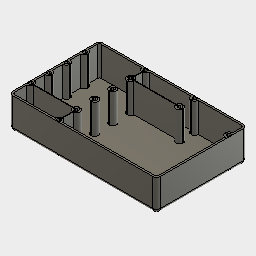
SIK_inserts v12 (Autodesk Fusion 360 design; units mm, degrees)
Autodesk Fusion 360 part; units mm, degrees
sketch "Sketch1" plane through (0, 0, 0) normal (0, 1, 0) x (1, 0, 0)
  line L0 (-107.65, -65.5) -> (133.65, -65.5)
  line L1 (140, -59.15) -> (140, 83.725)
  line L2 (133.65, 90.075) -> (-107.65, 90.075)
  line L3 (-114, 83.725) -> (-114, -59.15)
  arc A0 (-114, -59.15) -> (-107.65, -65.5) centre (-107.65, -59.15) ccw
  arc A1 (140, 83.725) -> (133.65, 90.075) centre (133.65, 83.725) ccw
  arc A2 (133.65, -65.5) -> (140, -59.15) centre (133.65, -59.15) ccw
  arc A3 (-107.65, 90.075) -> (-114, 83.725) centre (-107.65, 83.725) ccw
  point P0 (-114, -65.5)
  point P1 (140, -65.5)
  point P2 (-114, 90.075)
  dimension "d1" = 155.575
  dimension "d2" = 254
  dimension "d3" = 6.35
  dimension "d4" = 6.35
  dimension "d5" = 6.35
  dimension "d6" = 6.35
  measures "d1" distance of P0 P2
  measures "d2" distance of P0 P1
  measures "d3" radius of A0
  measures "d4" radius of A1
  measures "d5" radius of A2
  measures "d6" radius of A3
extrude "Extrude1" add sketch "Sketch1" along normal blind 3.175
sketch "Sketch2" plane through (0, 3.175, 0) normal (0, 1, 0) x (-1, 0, 0)
  arc A0 (107.65, -90.075) -> (114, -83.725) centre (107.65, -83.725) ccw
  line L0 (114, -83.725) -> (114, 59.15)
  arc A1 (114, 59.15) -> (107.65, 65.5) centre (107.65, 59.15) ccw
  line L1 (107.65, 65.5) -> (-133.65, 65.5)
  arc A2 (-133.65, 65.5) -> (-140, 59.15) centre (-133.65, 59.15) ccw
  line L2 (-140, 59.15) -> (-140, -83.725)
  arc A3 (-140, -83.725) -> (-133.65, -90.075) centre (-133.65, -83.725) ccw
  line L3 (-133.65, -90.075) -> (107.65, -90.075)
  line L4 (-136.825, 59.15) -> (-136.825, -83.725)
  arc A4 (-136.825, -83.725) -> (-133.65, -86.9) centre (-133.65, -83.725) ccw
  line L5 (-133.65, -86.9) -> (107.65, -86.9)
  arc A5 (107.65, -86.9) -> (110.825, -83.725) centre (107.65, -83.725) ccw
  line L6 (110.825, -83.725) -> (110.825, 59.15)
  arc A6 (110.825, 59.15) -> (107.65, 62.325) centre (107.65, 59.15) ccw
  line L7 (107.65, 62.325) -> (-133.65, 62.325)
  arc A7 (-133.65, 62.325) -> (-136.825, 59.15) centre (-133.65, 59.15) ccw
  circle A8 centre (31.45, 62.325) radius 3.175
  circle A9 centre (-136.825, -61.5) radius 3.175
  circle A10 centre (31.45, -61.5) radius 3.175
  circle A11 centre (31.45, -86.9) radius 3.175
  circle A12 centre (110.825, -61.5) radius 3.175
  circle A13 centre (31.45, 31.3688) radius 3.175
  circle A14 centre (31.45, 0.4125) radius 3.175
  circle A15 centre (31.45, -30.5437) radius 3.175
  circle A16 centre (-52.6875, -61.5) radius 3.175
  circle A17 centre (-52.6875, -86.9) radius 3.175
  circle A18 centre (110.825, -30.5437) radius 3.175
  circle A19 centre (110.825, 0.4125) radius 3.175
  circle A20 centre (110.825, 31.3688) radius 3.175
  circle A21 centre (31.45, 62.325) radius 6.35
  circle A22 centre (31.45, 31.3688) radius 6.35
  circle A23 centre (31.45, 0.4125) radius 6.35
  circle A24 centre (110.825, 31.3688) radius 6.35
  circle A25 centre (110.825, 0.4125) radius 6.35
  circle A26 centre (31.45, -30.5437) radius 6.35
  circle A27 centre (110.825, -30.5437) radius 6.35
  circle A28 centre (110.825, -61.5) radius 6.35
  circle A29 centre (31.45, -61.5) radius 6.35
  circle A30 centre (31.45, -86.9) radius 6.35
  circle A31 centre (-52.6875, -86.9) radius 6.35
  circle A32 centre (-52.6875, -61.5) radius 6.35
  circle A33 centre (-136.825, -61.5) radius 6.35
  line L8 (31.45, 31.3688) -> (110.825, 31.3688)
  line L9 (31.45, 0.4125) -> (110.825, 0.4125)
  line L10 (31.45, -30.5437) -> (110.825, -30.5437)
  line L11 (31.45, -61.5) -> (110.825, -61.5)
  line L12 (-52.6875, -61.5) -> (31.45, -61.5)
  line L13 (-136.825, -61.5) -> (-52.6875, -61.5)
  line L14 (-52.6875, -86.9) -> (-52.6875, -61.5)
  line L15 (31.45, -86.9) -> (31.45, -61.5)
  line L16 (31.45, -61.5) -> (31.45, -30.5437)
  line L17 (31.45, 0.4125) -> (31.45, -30.5437)
  line L18 (31.45, 31.3688) -> (31.45, 0.4125)
  line L19 (31.45, 62.325) -> (31.45, 31.3688)
  line L20 (31.45, 62.325) -> (31.45, 31.3688)
  line L21 (30.45, 62.325) -> (30.45, 31.3688)
  line L22 (31.45, 62.325) -> (31.45, 31.3688)
  line L23 (31.45, 62.325) -> (31.45, 31.3688)
  line L24 (32.45, 62.325) -> (32.45, 31.3688)
  line L25 (32.45, 31.3688) -> (32.45, 0.4125)
  line L26 (30.45, 31.3688) -> (30.45, 0.4125)
  line L27 (32.45, 0.4125) -> (32.45, -30.5437)
  line L28 (30.45, 0.4125) -> (30.45, -33.5572)
  line L29 (32.45, -30.5437) -> (32.45, -61.5)
  line L30 (30.45, -31.6976) -> (30.45, -61.5)
  line L31 (32.45, -61.5) -> (32.45, -86.9)
  line L32 (30.45, -61.5) -> (30.45, -86.9)
  line L33 (31.45, 30.3688) -> (110.825, 30.3688)
  line L34 (31.45, 31.3688) -> (110.825, 31.3688)
  line L35 (31.45, 32.3688) -> (110.825, 32.3688)
  line L36 (31.45, -0.5875) -> (110.825, -0.5875)
  line L37 (31.45, 0.4125) -> (110.825, 0.4125)
  line L38 (31.45, 1.4125) -> (110.825, 1.4125)
  line L39 (31.45, -31.5437) -> (110.825, -31.5437)
  line L40 (31.45, -30.5437) -> (110.825, -30.5437)
  line L41 (31.45, -29.5437) -> (110.825, -29.5437)
  line L42 (110.825, -61.5) -> (31.45, -61.5)
  line L43 (110.825, -60.5) -> (31.45, -60.5)
  line L44 (110.825, -62.5) -> (31.45, -62.5)
  line L45 (31.45, -62.5) -> (-136.825, -62.5)
  line L46 (31.45, -60.5) -> (-136.825, -60.5)
  line L47 (-52.6875, -61.5) -> (-52.6875, -86.9)
  line L48 (-51.6875, -86.9) -> (-51.6875, -61.5)
  line L49 (-53.6875, -86.9) -> (-53.6875, -61.5)
  line L50 (-133.65, -88.575) -> (107.65, -88.575)
  arc A34 (107.65, -88.575) -> (112.5, -83.725) centre (107.65, -83.725) ccw
  line L51 (112.5, -83.725) -> (112.5, 59.15)
  arc A35 (112.5, 59.15) -> (107.65, 64) centre (107.65, 59.15) ccw
  line L52 (107.65, 64) -> (-133.65, 64)
  arc A36 (-133.65, 64) -> (-138.5, 59.15) centre (-133.65, 59.15) ccw
  line L53 (-138.5, 59.15) -> (-138.5, -83.725)
  arc A37 (-138.5, -83.725) -> (-133.65, -88.575) centre (-133.65, -83.725) ccw
  line L54 (-136.825, -61.5) -> (-134.5799, -63.7451)
  line L55 (-136.825, -61.5) -> (-133.65, -61.5) construction
  line L56 (-136.825, -61.5) -> (-139.0701, -59.2549)
  line L57 (-136.825, -61.5) -> (-133.65, -61.5) construction
  line L58 (-136.825, -61.5) -> (-139.0701, -63.7451)
  line L59 (-136.825, -61.5) -> (-134.5799, -59.2549)
  line L60 (-136.4714, -61.8536) -> (-134.2264, -59.6085)
  line L61 (-136.4714, -61.8536) -> (-138.7165, -64.0986)
  line L62 (-139.0701, -63.7451) -> (-134.5799, -59.2549)
  line L63 (-139.4236, -63.3915) -> (-134.9335, -58.9014)
  line L64 (-136.4714, -61.1464) -> (-134.2264, -63.3915)
  line L65 (-136.4714, -61.1464) -> (-138.7165, -58.9014)
  line L66 (-134.5799, -63.7451) -> (-139.0701, -59.2549)
  line L67 (-134.9335, -64.0986) -> (-139.4236, -59.6085)
  line L68 (-136.4714, -61.8536) -> (-138.7165, -64.0986)
  line L69 (-139.4236, -63.3915) -> (-134.9335, -58.9014)
  line L70 (-136.4714, -61.1464) -> (-138.7165, -58.9014)
  line L71 (-136.4714, -61.8536) -> (-134.2264, -59.6085)
  line L72 (-136.4714, -61.1464) -> (-134.2264, -63.3915)
  circle A38 centre (-136.825, -61.5) radius 3.175
  line L73 (-50.796, -64.0986) -> (-55.2861, -59.6085)
  line L74 (-52.3339, -61.1464) -> (-54.579, -58.9014)
  line L75 (-52.3339, -61.1464) -> (-50.0889, -63.3915)
  line L76 (-52.3339, -61.8536) -> (-54.579, -64.0986)
  line L77 (-55.2861, -63.3915) -> (-50.796, -58.9014)
  line L78 (-52.3339, -61.8536) -> (-50.0889, -59.6085)
  circle A39 centre (-52.6875, -61.5) radius 3.175
  line L79 (-55.2861, -88.7915) -> (-50.796, -84.3014)
  line L80 (-52.3339, -87.2536) -> (-54.579, -89.4986)
  circle A40 centre (-52.6875, -86.9) radius 3.175
  line L81 (-50.796, -89.4986) -> (-55.2861, -85.0085)
  line L82 (-52.3339, -86.5464) -> (-50.0889, -88.7915)
  line L83 (-52.3339, -87.2536) -> (-50.0889, -85.0085)
  line L84 (-52.3339, -86.5464) -> (-54.579, -84.3014)
  line L85 (28.8514, -63.3915) -> (33.3415, -58.9014)
  line L86 (31.8036, -61.8536) -> (29.5585, -64.0986)
  circle A41 centre (31.45, -61.5) radius 3.175
  line L87 (33.3415, -64.0986) -> (28.8514, -59.6085)
  line L88 (31.8036, -61.1464) -> (34.0486, -63.3915)
  line L89 (31.8036, -61.8536) -> (34.0486, -59.6085)
  line L90 (31.8036, -61.1464) -> (29.5585, -58.9014)
  line L91 (28.8514, -88.7915) -> (33.3415, -84.3014)
  line L92 (31.8036, -87.2536) -> (29.5585, -89.4986)
  circle A42 centre (31.45, -86.9) radius 3.175
  line L93 (33.3415, -89.4986) -> (28.8514, -85.0085)
  line L94 (31.8036, -86.5464) -> (34.0486, -88.7915)
  line L95 (31.8036, -87.2536) -> (34.0486, -85.0085)
  line L96 (31.8036, -86.5464) -> (29.5585, -84.3014)
  line L97 (108.2264, -63.3915) -> (112.7165, -58.9014)
  line L98 (111.1786, -61.8536) -> (108.9335, -64.0986)
  circle A43 centre (110.825, -61.5) radius 3.175
  line L99 (112.7165, -64.0986) -> (108.2264, -59.6085)
  line L100 (111.1786, -61.1464) -> (113.4236, -63.3915)
  line L101 (111.1786, -61.8536) -> (113.4236, -59.6085)
  line L102 (111.1786, -61.1464) -> (108.9335, -58.9014)
  line L103 (28.8514, -32.4353) -> (33.3415, -27.9451)
  line L104 (31.8036, -30.8973) -> (29.5585, -33.1424)
  circle A44 centre (31.45, -30.5437) radius 3.175
  line L105 (33.3415, -33.1424) -> (28.8514, -28.6522)
  line L106 (31.8036, -30.1902) -> (34.0486, -32.4353)
  line L107 (31.8036, -30.8973) -> (34.0486, -28.6522)
  line L108 (31.8036, -30.1902) -> (29.5585, -27.9451)
  line L109 (28.8514, -1.479) -> (33.3415, 3.0111)
  line L110 (31.8036, 0.0589) -> (29.5585, -2.1861)
  circle A45 centre (31.45, 0.4125) radius 3.175
  line L111 (33.3415, -2.1861) -> (28.8514, 2.304)
  line L112 (31.8036, 0.7661) -> (34.0486, -1.479)
  line L113 (31.8036, 0.0589) -> (34.0486, 2.304)
  line L114 (31.8036, 0.7661) -> (29.5585, 3.0111)
  line L115 (108.2264, -32.4353) -> (112.7165, -27.9451)
  line L116 (111.1786, -30.8973) -> (108.9335, -33.1424)
  circle A46 centre (110.825, -30.5437) radius 3.175
  line L117 (112.7165, -33.1424) -> (108.2264, -28.6522)
  line L118 (111.1786, -30.1902) -> (113.4236, -32.4353)
  line L119 (111.1786, -30.8973) -> (113.4236, -28.6522)
  line L120 (111.1786, -30.1902) -> (108.9335, -27.9451)
  line L121 (108.2264, -1.479) -> (112.7165, 3.0111)
  line L122 (111.1786, 0.0589) -> (108.9335, -2.1861)
  circle A47 centre (110.825, 0.4125) radius 3.175
  line L123 (112.7165, -2.1861) -> (108.2264, 2.304)
  line L124 (111.1786, 0.7661) -> (113.4236, -1.479)
  line L125 (111.1786, 0.0589) -> (113.4236, 2.304)
  line L126 (111.1786, 0.7661) -> (108.9335, 3.0111)
  line L127 (28.8514, 29.4772) -> (33.3415, 33.9674)
  line L128 (31.8036, 31.0152) -> (29.5585, 28.7701)
  circle A48 centre (31.45, 31.3688) radius 3.175
  line L129 (33.3415, 28.7701) -> (28.8514, 33.2603)
  line L130 (31.8036, 31.7223) -> (34.0486, 29.4772)
  line L131 (31.8036, 31.0152) -> (34.0486, 33.2603)
  line L132 (31.8036, 31.7223) -> (29.5585, 33.9674)
  line L133 (108.2264, 29.4772) -> (112.7165, 33.9674)
  line L134 (111.1786, 31.0152) -> (108.9335, 28.7701)
  circle A49 centre (110.825, 31.3688) radius 3.175
  line L135 (112.7165, 28.7701) -> (108.2264, 33.2603)
  line L136 (111.1786, 31.7223) -> (113.4236, 29.4772)
  line L137 (111.1786, 31.0152) -> (113.4236, 33.2603)
  line L138 (111.1786, 31.7223) -> (108.9335, 33.9674)
  line L139 (28.8514, 60.4335) -> (33.3415, 64.9236)
  line L140 (31.8036, 61.9714) -> (29.5585, 59.7264)
  circle A50 centre (31.45, 62.325) radius 3.175
  line L141 (33.3415, 59.7264) -> (28.8514, 64.2165)
  line L142 (31.8036, 62.6786) -> (34.0486, 60.4335)
  line L143 (31.8036, 61.9714) -> (34.0486, 64.2165)
  line L144 (31.8036, 62.6786) -> (29.5585, 64.9236)
  point P0 (31.45, -61.5)
  dimension "d9" = 3.175
  dimension "d12" = 165.1
  dimension "d13" = 120.65
  dimension "d14" = 6.35
  dimension "d15" = 6.35
  dimension "d18" = 6.35
  dimension "d19" = 6.35
  dimension "d20" = 6.35
  dimension "d21" = 6.35
  dimension "d22" = 6.35
  dimension "d23" = 6.35
  dimension "d24" = 6.35
  dimension "d25" = 6.35
  dimension "d26" = 6.35
  dimension "d27" = 6.35
  dimension "d28" = 6.35
  dimension "d29" = 3.175
  dimension "d30" = 3.175
  dimension "d31" = 3.175
  dimension "d32" = 3.175
  dimension "d33" = 3.175
  dimension "d34" = 3.175
  dimension "d35" = 3.175
  dimension "d36" = 3.175
  dimension "d37" = 3.175
  dimension "d38" = 3.175
  dimension "d39" = 3.175
  dimension "d40" = 3.175
  dimension "d41" = 3.175
  dimension "d42" = 1
  dimension "d43" = 1
  dimension "d44" = 1
  dimension "d45" = 1
  dimension "d46" = 1
  dimension "d47" = 1
  dimension "d48" = 1
  dimension "d49" = 1
  dimension "d50" = 1
  dimension "d51" = 1
  dimension "d52" = 1
  dimension "d53" = 1
  dimension "d54" = 1.5
  dimension "d58" = 45
  dimension "d59" = 135
  dimension "d60" = 0.5
  dimension "d61" = 0.5
  dimension "d62" = 0.5
  dimension "d63" = 0.5
  dimension "d64" = 6.35
  dimension "d65" = 6.35
  dimension "d66" = 6.35
  dimension "d67" = 6.35
  dimension "d68" = 6.35
  dimension "d69" = 6.35
  dimension "d70" = 6.35
  dimension "d71" = 6.35
  dimension "d72" = 6.35
  dimension "d73" = 6.35
  dimension "d74" = 6.35
  dimension "d75" = 6.35
  dimension "d76" = 6.35
  measures "d12" distance of L7.end A8.centre
  measures "d13" distance of L4.start A9.centre
  measures "d14" diameter of A8
  measures "d15" diameter of A9
  measures "d18" diameter of A10
  measures "d19" diameter of A11
  measures "d20" diameter of A12
  measures "d21" diameter of A13
  measures "d22" diameter of A14
  measures "d23" diameter of A15
  measures "d24" diameter of A16
  measures "d25" diameter of A17
  measures "d26" diameter of A18
  measures "d27" diameter of A19
  measures "d28" diameter of A20
  measures "d29" distance of A8
  measures "d30" distance of A13
  measures "d31" distance of A14
  measures "d32" distance of A20
  measures "d33" distance of A19
  measures "d34" distance of A15
  measures "d35" distance of A18
  measures "d36" distance of A12
  measures "d37" distance of A10
  measures "d38" distance of A11
  measures "d39" distance of A17
  measures "d40" distance of A16
  measures "d41" distance of A9
  measures "d58" angle of L54 L55
  measures "d59" angle of L56 L57
  measures "d64" diameter of A38
  measures "d65" diameter of A39
  measures "d66" diameter of A40
  measures "d67" diameter of A41
  measures "d68" diameter of A42
  measures "d69" diameter of A43
  measures "d70" diameter of A44
  measures "d71" diameter of A45
  measures "d72" diameter of A46
  measures "d73" diameter of A47
  measures "d74" diameter of A48
  measures "d75" diameter of A49
  measures "d76" diameter of A50
extrude "Extrude2" add sketch "Sketch2" along normal blind 50.8 contours A0 L0 L3 A28 A30 L50 A34 L51 | L3 A11 A30 L50 A42 | L0 A12 A28 L51 A43 | L3 A11 A30 L50 A42 | A11 L50 L92 A42 L93 | L3 A30 A31 L50 | L5 A11 A30 L50 A42 | L5 A5 L6 A28 A30 L50 A34 L51 | L0 A12 A28 L51 A43 | A12 L51 A43 L100 L101 | L6 A12 A28 L51 A43 | A11 L50 L91 L92 A42 | A11 L50 A42 L93 L94 | L3 A17 A31 L50 A40 | L5 A30 A31 L50 | L5 A11 A30 L50 A42 | L5 A11 A30 L31 A42 | A11 L50 A42 L94 | L0 A27 A28 L51 | A12 L51 L97 A43 L101 | A12 L51 A43 L99 L100 | L6 A12 A28 L44 A43 | A12 L51 A43 L99 | A11 L50 L91 A42 | L3 A17 A31 L50 A40 | A17 L50 L80 A40 L81 | L2 A3 L3 A31 A33 L50 L53 A37 | L5 A17 A31 L50 A40 | L5 A11 A30 L32 A42 | L0 A18 A27 L51 A46 | L6 A12 A28 L51 A43 | L6 A27 A28 L51 | A12 L51 L97 A43 | A17 L50 L79 L80 A40 | A17 L50 A40 L81 L82 | L4 A4 L5 A31 A33 L50 L53 A37 | L5 A17 A31 L50 A40 | L5 A17 A31 L48 A40 | A17 L50 A40 L82 | A10 A29 L31 L44 A41 | L0 A18 A27 L51 A46 | A18 L51 A46 L118 L119 | L6 A18 A27 L51 A46 | L6 A12 A28 L43 A43 | A17 L50 L79 A40 | L5 A17 A31 L49 A40 | A10 A29 L32 L45 A41 | L0 A25 A27 L51 | A18 L51 L115 A46 L119 | A18 L51 A46 L117 L118 | L6 A18 A27 L39 A46 | A18 L51 A46 L117 | L2 A9 A33 L53 A38 | A16 A32 L45 L48 A39 | L0 A19 A25 L51 A47 | L6 A18 A27 L51 A46 | L6 A25 A27 L51 | A18 L51 L115 A46 | A10 A29 L29 L43 A41 | L2 A9 A33 L53 A38 | A9 L53 L63 L67 L69 A38 | L1 A2 L2 A21 A33 L52 A36 L53 | L4 A9 A33 L53 A38 | A16 A32 L45 L49 A39 | L0 A19 A25 L51 A47 | A19 L51 A47 L124 L125 | L6 A19 A25 L51 A47 | L6 A18 A27 L41 A46 | A15 A26 L29 L39 A44 | A9 L53 L56 L66 L67 A38 | A9 L53 L58 L62 L63 L69 A38 | L4 L7 A7 A21 A33 L52 A36 L53 | L4 A9 A33 L53 A38 | L4 A9 A33 L45 A38 | A9 L53 L61 L68 A38 | A10 A29 L30 L46 A41 | L0 A24 A25 L51 | A19 L51 L121 A47 L125 | A19 L51 A47 L123 L124 | L6 A19 A25 L36 A47 | A19 L51 A47 L123 | A9 L53 L56 L65 L66 L70 A38 | A9 L53 L58 L61 L62 L68 A38 | L4 A9 A33 L46 A38 | A9 L53 L65 L70 A38 | A16 A32 L46 A39 | L0 A20 A24 L51 A49 | L6 A19 A25 L51 A47 | L6 A24 A25 L51 | A19 L51 L121 A47 | A15 A26 L27 L41 A44 | L1 A8 A21 L52 A50 | A15 A26 L28 L30 A44 | L0 A20 A24 L51 A49 | A20 L51 A49 L136 L137 | L6 A20 A24 L51 A49 | L6 A19 A25 L38 A47 | A14 A23 L27 L36 A45 | L1 A8 A21 L52 A50 | A8 L52 L139 A50 L144 | L0 A1 L1 A21 A24 L51 A35 L52 | L7 A8 A21 L52 A50 | A20 L51 L133 A49 L137 | A20 L51 A49 L135 L136 | L6 A20 A24 L33 A49 | A20 L51 A49 L135 | A8 L52 L139 A50 L143 | A8 L52 A50 L141 L144 | L6 A6 L7 A21 A24 L51 A35 L52 | L7 A8 A21 L52 A50 | L7 A8 A21 L21 A50 | A8 L52 A50 L141 | A14 A23 L26 L28 A45 | L6 A20 A24 L51 A49 | A20 L51 L133 A49 | A14 A23 L25 L38 A45 | A8 L52 A50 L143 | L7 A8 A21 L24 A50 | L6 A20 A24 L35 A49 | A13 A22 L25 L33 A48 | A13 A22 L21 L26 A48 | A13 A22 L24 L35 A48
fillet "Fillet1" radius 6.35 8 edges at (140, 0, -12.2875) (138.1401, 0, -88.2151) (13, 0, -90.075) (-112.1401, 0, -88.2151) (-114, 0, -12.2875) (-112.1401, 0, 63.6401) (13, 0, 65.5) (138.1401, 0, 63.6401)
sketch "split_break_dividers" plane through (0, 3.175, -3.175) normal (0, 1, 0) x (1, 0, 0)
  arc A0 (-32.45, -28.273) -> (-37.7208, -33.5438) centre (-31.45, -34.5438) ccw
  line L0 (50.6268, 57.6786) -> (50.226, 57.2777)
  arc A1 (50.226, 57.2777) -> (50.0596, 57.825) centre (52.6875, 58.325) cw
  line L1 (-107.65, 83.725) -> (133.65, 83.725)
  line L2 (134.5799, 60.5701) -> (139.0701, 56.0799)
  line L3 (-111.1786, 27.0152) -> (-108.9335, 24.7701)
  line L4 (136.4714, 58.6786) -> (134.2264, 56.4335)
  line L5 (-31.8036, 58.6786) -> (-34.0486, 56.4335)
  line L6 (-31.8036, 57.9714) -> (-34.0486, 60.2165)
  line L7 (52.3339, 83.3714) -> (54.579, 81.1264)
  line L8 (136.4714, 58.6786) -> (134.2264, 56.4335)
  line L9 (133.65, -67.175) -> (-107.65, -67.175)
  line L10 (-31.8036, -3.9411) -> (-29.5585, -6.1861)
  line L11 (51.2733, 58.325) -> (50.6268, 57.6786)
  line L12 (-28.8514, -1.696) -> (-33.3415, -6.1861)
  line L13 (-31.8036, 27.0152) -> (-34.0486, 29.2603)
  line L14 (-112.5, -62.325) -> (-112.5, 80.55)
  line L15 (-107.65, 86.9) -> (133.65, 86.9)
  arc A2 (136.825, -62.325) -> (133.65, -65.5) centre (133.65, -62.325) cw
  arc A3 (-28.8221, 57.825) -> (-28.9885, 57.2777) centre (-31.45, 58.325) cw
  line L16 (55.2861, 60.2165) -> (50.796, 55.7264)
  line L17 (-31.8036, 27.0152) -> (-29.5585, 24.7701)
  line L18 (-31.8036, -3.2339) -> (-29.5585, -0.9889)
  line L19 (140, 80.55) -> (140, -62.325)
  line L20 (-114, -62.325) -> (-114, 80.55)
  arc A4 (-107.65, -65.5) -> (-110.825, -62.325) centre (-107.65, -62.325) cw
  line L21 (-108.2264, 29.2603) -> (-112.7165, 24.7701)
  line L22 (50.796, 60.9236) -> (55.2861, 56.4335)
  line L23 (52.3339, 83.3714) -> (50.0889, 85.6165)
  line L24 (-31.8036, -3.2339) -> (-34.0486, -5.479)
  line L25 (133.65, -65.5) -> (-107.65, -65.5)
  line L26 (-33.3415, 29.9674) -> (-28.8514, 25.4772)
  line L27 (133.65, -68.675) -> (-107.65, -68.675)
  line L28 (-31.8036, 27.7223) -> (-34.0486, 25.4772)
  line L29 (-31.8036, -3.9411) -> (-34.0486, -1.696)
  line L30 (-33.3415, -0.9889) -> (-28.8514, -5.479)
  line L31 (55.2861, 85.6165) -> (50.796, 81.1264)
  line L32 (136.4714, 57.9714) -> (134.2264, 60.2165)
  line L33 (-107.65, 85.4) -> (133.65, 85.4)
  arc A5 (-107.65, -67.175) -> (-112.5, -62.325) centre (-107.65, -62.325) cw
  arc A6 (133.65, 83.725) -> (136.825, 80.55) centre (133.65, 80.55) cw
  arc A7 (-110.825, 80.55) -> (-107.65, 83.725) centre (-107.65, 80.55) cw
  line L34 (136.825, 80.55) -> (136.825, -62.325)
  arc A8 (140, -62.325) -> (133.65, -68.675) centre (133.65, -62.325) cw
  line L35 (52.3339, 58.6786) -> (54.579, 60.9236)
  line L36 (-111.1786, 27.7223) -> (-113.4236, 25.4772)
  line L37 (-111.1786, 58.6786) -> (-113.4236, 56.4335)
  line L38 (136.825, 58.325) -> (134.5799, 60.5701)
  line L39 (-110.825, -62.325) -> (-110.825, 80.55)
  arc A9 (-114, 80.55) -> (-107.65, 86.9) centre (-107.65, 80.55) cw
  line L40 (136.825, 58.325) -> (136.1179, 58.325)
  arc A10 (-107.65, -68.675) -> (-114, -62.325) centre (-107.65, -62.325) cw
  line L41 (136.4714, 57.9714) -> (134.2264, 60.2165)
  arc A11 (-112.5, 80.55) -> (-107.65, 85.4) centre (-107.65, 80.55) cw
  line L42 (50.6268, 58.9714) -> (51.2733, 58.325)
  line L43 (52.3339, 57.9714) -> (54.579, 55.7264)
  line L44 (-112.7165, 60.9236) -> (-108.2264, 56.4335)
  arc A12 (138.5, -62.325) -> (133.65, -67.175) centre (133.65, -62.325) cw
  line L45 (138.5, 80.55) -> (138.5, -62.325)
  line L46 (50.0596, 57.825) -> (-28.8221, 57.825)
  line L47 (136.4714, 57.9714) -> (138.7165, 55.7264)
  arc A13 (133.65, 85.4) -> (138.5, 80.55) centre (133.65, 80.55) cw
  arc A14 (133.65, 86.9) -> (140, 80.55) centre (133.65, 80.55) cw
  line L48 (-111.1786, 27.7223) -> (-108.9335, 29.9674)
  line L49 (139.0701, 60.5701) -> (134.5799, 56.0799)
  line L50 (-111.1786, 27.0152) -> (-113.4236, 29.2603)
  arc A15 (-34.0779, -35.0438) -> (-33.9115, -35.591) centre (-31.45, -34.5438) ccw
  line L51 (-109.1179, -33.5438) -> (-110.1179, -34.5438)
  line L52 (-29.5865, 60.8956) -> (-29.5585, 60.9236)
  line L53 (-34.0206, -36.4072) -> (-34.0486, -36.4353)
  line L54 (-108.1971, -35.0438) -> (-34.0779, -35.0438)
  line L55 (-30.45, 60.0321) -> (-29.5865, 60.8956)
  line L56 (-33.3415, 60.9236) -> (-33.3135, 60.8956)
  line L57 (-33.5107, -33.8973) -> (-33.9115, -33.4965)
  line L58 (-33.3135, -31.9731) -> (-31.45, -33.8366)
  line L59 (-31.45, -33.8366) -> (-28.8514, -36.4353)
  line L60 (-33.1571, -33.5438) -> (-34.0206, -32.6803)
  line L61 (-32.8642, -34.5438) -> (-33.5107, -33.8973)
  line L62 (-33.1571, -35.5438) -> (-34.0206, -36.4072)
  line L63 (-33.5107, -35.1902) -> (-32.8642, -34.5438)
  line L64 (-31.1571, 59.325) -> (-30.45, 60.0321)
  line L65 (50.1169, 60.1885) -> (50.0889, 60.2165)
  line L66 (50.9804, 59.325) -> (50.1169, 60.1885)
  line L67 (51.6875, 58.6179) -> (50.9804, 59.325)
  arc A16 (49.6741, 57.325) -> (50.1169, 56.4615) centre (52.6875, 58.325) ccw
  line L68 (-32.45, 82.0179) -> (-33.3135, 81.1544)
  arc A17 (50.1169, 60.1885) -> (49.6741, 59.325) centre (52.6875, 58.325) ccw
  line L69 (-28.9885, 57.2777) -> (-29.3893, 57.6786)
  line L70 (-28.8794, 56.4615) -> (-28.8514, 56.4335)
  line L71 (-110.1179, -34.5438) -> (-112.7165, -37.1424)
  line L72 (-108.2544, -36.4072) -> (-108.2264, -36.4353)
  line L73 (-108.2264, -32.6522) -> (-108.2544, -32.6803)
  line L74 (-112.7165, -31.9451) -> (-110.1179, -34.5438)
  arc A18 (-107.8116, -33.5438) -> (-108.2544, -32.6803) centre (-110.825, -34.5438) ccw
  arc A19 (-34.4634, -35.5438) -> (-34.0206, -36.4072) centre (-31.45, -34.5438) ccw
  arc A20 (-108.3635, -35.591) -> (-108.1971, -35.0438) centre (-110.825, -34.5438) ccw
  line L75 (-34.0206, -32.6803) -> (-34.0486, -32.6522)
  line L76 (-33.9115, -35.591) -> (-33.5107, -35.1902)
  arc A21 (-33.9115, -33.4965) -> (-34.0779, -34.0438) centre (-31.45, -34.5438) ccw
  arc A22 (-32.45, -31.5303) -> (-33.3135, -31.9731) centre (-31.45, -34.5438) ccw
  line L77 (-108.2544, -32.6803) -> (-109.1179, -33.5438)
  line L78 (-108.7643, -35.1902) -> (-108.3635, -35.591)
  line L79 (-30.7429, 58.325) -> (-30.45, 58.0321)
  arc A23 (-32.4973, 60.7865) -> (-31.95, 60.9529) centre (-31.45, 58.325) cw
  arc A24 (-108.1971, -34.0438) -> (-108.3635, -33.4965) centre (-110.825, -34.5438) ccw
  line L80 (-110.1179, -34.5438) -> (-109.1179, -35.5438)
  line L81 (-109.1179, -35.5438) -> (-108.2544, -36.4072)
  line L82 (-34.0779, -34.0438) -> (-108.1971, -34.0438)
  line L83 (-32.45, -34.2509) -> (-33.1571, -33.5438)
  line L84 (-108.3635, -33.4965) -> (-108.7643, -33.8973)
  line L85 (-109.4108, -34.5438) -> (-108.7643, -35.1902)
  arc A25 (-108.2544, -36.4072) -> (-107.8116, -35.5438) centre (-110.825, -34.5438) ccw
  line L86 (-33.3415, -31.9451) -> (-33.3135, -31.9731)
  line L87 (-32.45, -34.8366) -> (-33.1571, -35.5438)
  line L88 (-108.7643, -33.8973) -> (-109.4108, -34.5438)
  line L89 (51.9804, 58.325) -> (50.9804, 57.325)
  line L90 (-33.3135, 81.1544) -> (-33.3415, 81.1264)
  line L91 (-31.45, 83.0179) -> (-32.45, 82.0179)
  arc A26 (-33.3135, 81.1544) -> (-32.45, 80.7116) centre (-31.45, 83.725) ccw
  line L92 (-30.0358, 58.325) -> (-29.3893, 58.9714)
  arc A27 (50.0596, 58.825) -> (50.226, 59.3723) centre (52.6875, 58.325) cw
  line L93 (-30.4027, 60.7865) -> (-30.8036, 60.3857)
  line L94 (50.9804, 57.325) -> (50.1169, 56.4615)
  line L95 (-31.8036, 83.3714) -> (-31.45, 83.0179)
  line L96 (52.3339, 57.9714) -> (51.9804, 58.325)
  line L97 (-30.45, 82.0179) -> (-29.5865, 81.1544)
  line L98 (50.226, 59.3723) -> (50.6268, 58.9714)
  line L99 (-28.8794, 60.1885) -> (-29.7429, 59.325)
  line L100 (-30.8036, 60.3857) -> (-31.45, 59.7392)
  line L101 (-31.95, 60.9529) -> (-31.95, 81.0971)
  arc A28 (-28.4366, 59.325) -> (-28.8794, 60.1885) centre (-31.45, 58.325) ccw
  line L102 (-31.45, 82.3108) -> (-30.8036, 81.6643)
  line L103 (-29.7429, 59.325) -> (-30.45, 58.6179)
  line L104 (-32.4973, 81.2635) -> (-32.0964, 81.6643)
  arc A29 (-30.4027, 81.2635) -> (-30.95, 81.0971) centre (-31.45, 83.725) cw
  line L105 (-29.5865, 81.1544) -> (-29.5585, 81.1264)
  line L106 (-33.3135, 60.8956) -> (-32.45, 60.0321)
  line L107 (-31.7429, 59.325) -> (-31.45, 59.0321)
  line L108 (-31.45, 59.0321) -> (-30.7429, 58.325)
  arc A30 (-29.5865, 60.8956) -> (-30.45, 61.3384) centre (-31.45, 58.325) ccw
  line L109 (-28.8514, 60.2165) -> (-28.8794, 60.1885)
  line L110 (-28.8514, 85.6165) -> (-31.45, 83.0179)
  arc A31 (-32.45, 61.3384) -> (-33.3135, 60.8956) centre (-31.45, 58.325) ccw
  arc A32 (-31.95, 81.0971) -> (-32.4973, 81.2635) centre (-31.45, 83.725) cw
  line L111 (-30.8036, 81.6643) -> (-30.4027, 81.2635)
  line L112 (51.9804, 58.325) -> (51.6875, 58.6179)
  line L113 (-29.3893, 57.6786) -> (-30.0358, 58.325)
  line L114 (-31.45, 59.7392) -> (-32.0964, 60.3857)
  line L115 (-29.7429, 57.325) -> (-28.8794, 56.4615)
  arc A33 (-28.8794, 56.4615) -> (-28.4366, 57.325) centre (-31.45, 58.325) ccw
  line L116 (-30.45, 58.0321) -> (-29.7429, 57.325)
  line L117 (-32.45, 60.0321) -> (-31.7429, 59.325)
  arc A34 (-30.95, 60.9529) -> (-30.4027, 60.7865) centre (-31.45, 58.325) cw
  line L118 (-31.45, 83.0179) -> (-30.45, 82.0179)
  line L119 (-31.45, 59.0321) -> (-31.1571, 59.325)
  line L120 (-32.0964, 81.6643) -> (-31.45, 82.3108)
  line L121 (-32.0964, 60.3857) -> (-32.4973, 60.7865)
  line L122 (52.3339, 58.6786) -> (51.9804, 58.325)
  arc A35 (-28.9885, 59.3723) -> (-28.8221, 58.825) centre (-31.45, 58.325) cw
  line L123 (-28.8221, 58.825) -> (50.0596, 58.825)
  line L124 (-29.3893, 58.9714) -> (-28.9885, 59.3723)
  line L125 (-31.8036, 58.6786) -> (-31.45, 59.0321)
  line L126 (-30.7429, 58.325) -> (-33.3415, 55.7264)
  arc A36 (-30.45, 80.7116) -> (-29.5865, 81.1544) centre (-31.45, 83.725) ccw
  line L127 (50.1169, 56.4615) -> (50.0889, 56.4335)
  line L128 (-30.45, 58.6179) -> (-30.7429, 58.325)
  line L129 (-30.95, 81.0971) -> (-30.95, 60.9529)
  line L130 (-31.45, -34.5438) -> (-32.1571, -34.5438)
  line L131 (-34.4634, -2.5875) -> (-107.8116, -2.5875)
  line L132 (-110.825, 58.325) -> (-110.1179, 58.325)
  line L133 (-34.4634, -35.5438) -> (-107.8116, -35.5438)
  arc A37 (-32.45, 33.6395) -> (-37.7208, 28.3687) centre (-31.45, 27.3687) ccw
  line L134 (-31.7429, -2.5875) -> (-33.1571, -2.5875)
  line L135 (-34.4634, 26.3687) -> (-107.8116, 26.3687)
  arc A38 (-37.7208, 26.3687) -> (-30.45, 33.6395) centre (-31.45, 27.3687) ccw
  line L136 (-32.45, -35.5438) -> (-33.1571, -35.5438)
  line L137 (-110.825, 59.325) -> (-109.1179, 59.325)
  arc A39 (-34.4634, -4.5875) -> (-32.45, -6.6009) centre (-31.45, -3.5875) ccw
  line L138 (-31.45, -3.5875) -> (-32.1571, -3.5875)
  arc A40 (-37.7208, -35.5438) -> (-32.45, -40.8145) centre (-31.45, -34.5438) ccw
  arc A41 (-107.8116, -2.5875) -> (-107.8116, -4.5875) centre (-110.825, -3.5875) ccw
  line L139 (-109.1179, -4.5875) -> (-110.825, -4.5875)
  arc A42 (-30.45, 80.7116) -> (-33.3135, 81.1544) centre (-31.45, 83.725) ccw
  arc A43 (-33.3135, -31.9731) -> (-34.0206, -32.6803) centre (-31.45, -34.5438) ccw
  line L140 (-32.45, -33.5438) -> (-33.1571, -33.5438)
  line L141 (-31.7429, 28.3687) -> (-33.1571, 28.3687)
  arc A44 (-34.4634, 26.3687) -> (-32.45, 24.3553) centre (-31.45, 27.3687) ccw
  arc A45 (-104.5542, 28.3687) -> (-104.5542, 26.3687) centre (-110.825, 27.3687) ccw
  line L142 (-34.4634, -33.5438) -> (-107.8116, -33.5438)
  arc A46 (-34.0206, -36.4072) -> (-33.3135, -37.1144) centre (-31.45, -34.5438) ccw
  arc A47 (-32.45, 2.6833) -> (-37.7208, -2.5875) centre (-31.45, -3.5875) ccw
  line L143 (-31.45, 27.3687) -> (-32.1571, 27.3687)
  arc A48 (-34.4634, 26.3687) -> (-32.45, 24.3553) centre (-31.45, 27.3687) ccw
  line L144 (-110.1179, 58.325) -> (-110.825, 58.325)
  line L145 (-31.45, -3.5875) -> (-32.1571, -3.5875)
  arc A49 (-29.5865, 81.1544) -> (-32.45, 80.7116) centre (-31.45, 83.725) ccw
  line L146 (-32.45, 82.0179) -> (-32.45, 83.725)
  line L147 (-109.1179, -33.5438) -> (-110.825, -33.5438)
  line L148 (-34.4634, -4.5875) -> (-107.8116, -4.5875)
  line L149 (-30.45, -62.4866) -> (-30.45, -37.5572)
  line L150 (-30.45, 56.6179) -> (-30.45, 58.0321)
  line L151 (-32.45, 30.3822) -> (-32.45, 55.3116)
  arc A50 (-30.45, -6.6009) -> (-30.45, -0.5741) centre (-31.45, -3.5875) ccw
  arc A51 (-30.45, -9.8583) -> (-30.45, 2.6833) centre (-31.45, -3.5875) ccw
  line L152 (-32.45, -62.4866) -> (-32.45, -37.5572)
  arc A52 (-30.45, -37.5572) -> (-30.45, -31.5303) centre (-31.45, -34.5438) ccw
  line L153 (-31.45, -3.5875) -> (-31.45, -2.8804)
  line L154 (-32.45, 27.6616) -> (-32.45, 29.0759)
  line L155 (-112.7165, -0.9889) -> (-108.2264, -5.479)
  arc A53 (-30.45, 24.3553) -> (-30.45, 30.3822) centre (-31.45, 27.3687) ccw
  line L156 (-111.1786, -34.8973) -> (-113.4236, -32.6522)
  line L157 (-111.1786, -3.9411) -> (-113.4236, -1.696)
  line L158 (-30.45, 28.5226) -> (-30.45, 29.0759)
  arc A54 (-33.3135, -62.9294) -> (-29.5865, -62.9294) centre (-31.45, -65.5) ccw
  line L159 (-31.8036, -65.8536) -> (-34.0486, -63.6085)
  line L160 (-32.45, 25.6616) -> (-32.45, 27.0759)
  arc A55 (-29.5865, -37.1144) -> (-29.5865, -31.9731) centre (-31.45, -34.5438) ccw
  line L161 (-32.45, 56.6179) -> (-32.45, 58.0321)
  arc A56 (-32.45, 30.3822) -> (-34.4634, 28.3687) centre (-31.45, 27.3687) ccw
  line L162 (-31.45, 59.0321) -> (-31.45, 58.325)
  line L163 (-112.7165, 29.9674) -> (-108.2264, 25.4772)
  line L164 (-111.1786, 57.9714) -> (-113.4236, 60.2165)
  line L165 (-33.3415, 86.3236) -> (-28.8514, 81.8335)
  line L166 (52.3339, 84.0786) -> (50.0889, 81.8335)
  line L167 (-31.8036, 57.9714) -> (-29.5585, 55.7264)
  line L168 (52.3339, 84.0786) -> (54.579, 86.3236)
  line L169 (-31.8036, 84.0786) -> (-34.0486, 81.8335)
  line L170 (134.9335, 60.9236) -> (139.4236, 56.4335)
  line L171 (136.825, 58.325) -> (134.5799, 56.0799)
  line L172 (-31.8036, 83.3714) -> (-34.0486, 85.6165)
  line L173 (-28.8514, 29.2603) -> (-33.3415, 24.7701)
  line L174 (139.4236, 60.2165) -> (134.9335, 55.7264)
  line L175 (136.4714, 58.6786) -> (138.7165, 60.9236)
  line L176 (136.825, 58.325) -> (136.1179, 58.325)
  line L177 (136.825, 58.325) -> (139.0701, 56.0799)
  line L178 (136.825, 58.325) -> (139.0701, 60.5701)
  line L179 (50.796, 86.3236) -> (55.2861, 81.8335)
  arc A57 (-32.45, -59.2292) -> (-30.45, -59.2292) centre (-31.45, -65.5) ccw
  line L180 (-31.8036, -65.8536) -> (-29.5585, -68.0986)
  line L181 (139.4236, 60.2165) -> (134.9335, 55.7264)
  line L182 (-111.1786, 58.6786) -> (-108.9335, 60.9236)
  line L183 (136.4714, 57.9714) -> (138.7165, 55.7264)
  line L184 (-108.2264, 60.2165) -> (-112.7165, 55.7264)
  line L185 (-32.45, -35.5438) -> (-32.45, -34.8366)
  line L186 (-31.8036, 84.0786) -> (-29.5585, 86.3236)
  line L187 (-31.8036, 27.7223) -> (-29.5585, 29.9674)
  line L188 (136.4714, 58.6786) -> (138.7165, 60.9236)
  line L189 (-111.1786, -34.8973) -> (-108.9335, -37.1424)
  line L190 (-32.45, 58.6179) -> (-32.45, 60.0321)
  line L191 (-30.45, 58.6179) -> (-30.45, 60.0321)
  line L192 (-111.1786, 57.9714) -> (-108.9335, 55.7264)
  line L193 (-32.45, 61.3384) -> (-32.45, 80.7116)
  arc A58 (-30.45, 24.3553) -> (-30.45, 30.3822) centre (-31.45, 27.3687) ccw
  line L194 (-30.45, -3.5875) -> (-30.45, -1.8804)
  line L195 (-30.45, -65.5) -> (-30.45, -65.2071)
  line L196 (-30.45, 61.3384) -> (-30.45, 80.7116)
  line L197 (-31.45, 58.325) -> (-31.45, 57.6179)
  line L198 (-111.1786, -34.1902) -> (-113.4236, -36.4353)
  line L199 (-108.2264, -1.696) -> (-112.7165, -6.1861)
  line L200 (-30.45, 30.3822) -> (-30.45, 55.3116)
  line L201 (-111.1786, -3.9411) -> (-108.9335, -6.1861)
  line L202 (-111.1786, -34.1902) -> (-108.9335, -31.9451)
  line L203 (-28.8514, -63.6085) -> (-33.3415, -68.0986)
  line L204 (-30.45, -5.2946) -> (-30.45, -3.5875)
  line L205 (-31.45, -34.5438) -> (-31.45, -33.8366)
  line L206 (-31.45, 83.725) -> (-31.45, 83.0179)
  line L207 (-32.45, -65.5) -> (-32.45, -65.2071)
  line L208 (-31.45, -65.5) -> (-31.45, -64.7929)
  line L209 (-32.45, -5.2946) -> (-32.45, -3.8804)
  line L210 (-30.45, 25.6616) -> (-30.45, 29.0759)
  line L211 (-31.8036, -65.1464) -> (-34.0486, -67.3915)
  arc A59 (-30.45, -6.6009) -> (-30.45, -0.5741) centre (-31.45, -3.5875) ccw
  arc A60 (-32.45, -62.4866) -> (-30.45, -62.4866) centre (-31.45, -65.5) ccw
  line L212 (-30.45, -34.8366) -> (-30.45, -34.5438)
  arc A61 (-30.45, -40.8145) -> (-30.45, -28.273) centre (-31.45, -34.5438) ccw
  line L213 (-32.45, -31.5303) -> (-32.45, -6.6009)
  line L214 (-31.45, 26.6616) -> (-31.45, 27.3687)
  line L215 (-32.45, -0.5741) -> (-32.45, 24.3553)
  line L216 (-30.45, -0.5741) -> (-30.45, 24.3553)
  line L217 (-32.45, -34.2509) -> (-32.45, -33.5438)
  line L218 (-31.45, -35.2509) -> (-31.45, -34.5438)
  line L219 (-30.45, -31.5303) -> (-30.45, -6.6009)
  line L220 (-31.45, -4.2946) -> (-31.45, -3.5875)
  line L221 (-31.45, 28.0759) -> (-31.45, 27.3687)
  line L222 (-30.45, 82.0179) -> (-30.45, 83.725)
  line L223 (-111.1786, -3.2339) -> (-113.4236, -5.479)
  line L224 (-111.1786, -3.2339) -> (-108.9335, -0.9889)
  line L225 (-32.45, -3.2946) -> (-32.45, -1.8804)
  line L226 (-30.45, -34.5438) -> (-30.45, -34.2509)
  arc A62 (58.9583, 59.325) -> (53.6875, 64.5958) centre (52.6875, 58.325) ccw
  arc A63 (-104.5542, 59.325) -> (-104.5542, 57.325) centre (-110.825, 58.325) ccw
  arc A64 (-30.45, 52.0542) -> (-25.1792, 57.325) centre (-31.45, 58.325) ccw
  arc A65 (-25.1792, 59.325) -> (-30.45, 64.5958) centre (-31.45, 58.325) ccw
  arc A66 (53.6875, 80.7116) -> (51.6875, 80.7116) centre (52.6875, 83.725) ccw
  line L227 (-31.45, 27.3687) -> (-32.1571, 27.3687)
  arc A67 (-32.45, 30.3822) -> (-34.4634, 28.3687) centre (-31.45, 27.3687) ccw
  arc A68 (50.1169, 56.4615) -> (55.7009, 57.325) centre (52.6875, 58.325) ccw
  line L228 (55.7009, 57.325) -> (133.8116, 57.325)
  line L229 (-110.1179, -34.5438) -> (-110.825, -34.5438)
  line L230 (52.6875, 83.0179) -> (52.6875, 83.725)
  arc A69 (-32.45, 64.5958) -> (-37.7208, 59.325) centre (-31.45, 58.325) ccw
  line L231 (-110.1179, 27.3687) -> (-110.825, 27.3687)
  line L232 (-33.1571, 57.325) -> (-31.7429, 57.325)
  line L233 (-109.1179, -35.5438) -> (-110.825, -35.5438)
  line L234 (51.6875, 80.7116) -> (51.6875, 61.3384)
  line L235 (-110.1179, -3.5875) -> (-110.825, -3.5875)
  line L236 (-31.45, -34.5438) -> (-32.1571, -34.5438)
  arc A70 (-32.45, -0.5741) -> (-34.4634, -2.5875) centre (-31.45, -3.5875) ccw
  arc A71 (-32.45, -31.5303) -> (-34.4634, -33.5438) centre (-31.45, -34.5438) ccw
  arc A72 (-107.8116, -2.5875) -> (-107.8116, -4.5875) centre (-110.825, -3.5875) ccw
  arc A73 (-107.8116, -33.5438) -> (-107.8116, -35.5438) centre (-110.825, -34.5438) ccw
  line L237 (-109.1179, 28.3687) -> (-110.825, 28.3687)
  line L238 (55.7009, 59.325) -> (133.8116, 59.325)
  arc A74 (-30.45, 55.3116) -> (-28.8794, 56.4615) centre (-31.45, 58.325) ccw
  line L239 (51.6875, 83.725) -> (51.6875, 82.0179)
  arc A75 (-34.4634, 57.325) -> (-32.45, 55.3116) centre (-31.45, 58.325) ccw
  arc A76 (-108.2544, -32.6803) -> (-108.2544, -36.4072) centre (-110.825, -34.5438) ccw
  line L240 (52.6875, 58.325) -> (51.9804, 58.325)
  arc A77 (133.8116, 57.325) -> (133.8116, 59.325) centre (136.825, 58.325) ccw
  line L241 (-110.1179, -3.5875) -> (-110.825, -3.5875)
  line L242 (-109.1179, 26.3687) -> (-110.825, 26.3687)
  line L243 (-110.1179, 27.3687) -> (-110.825, 27.3687)
  arc A78 (-104.5542, -2.5875) -> (-104.5542, -4.5875) centre (-110.825, -3.5875) ccw
  line L244 (52.9804, 59.325) -> (54.3946, 59.325)
  arc A79 (-32.45, 61.3384) -> (-34.4634, 59.325) centre (-31.45, 58.325) ccw
  line L245 (-110.825, 57.325) -> (-109.1179, 57.325)
  arc A80 (55.7009, 59.325) -> (53.6875, 61.3384) centre (52.6875, 58.325) ccw
  arc A81 (-34.0206, -36.4072) -> (-32.45, -37.5572) centre (-31.45, -34.5438) ccw
  arc A82 (133.8116, 57.325) -> (133.8116, 59.325) centre (136.825, 58.325) ccw
  arc A83 (-30.45, 55.3116) -> (-28.4366, 57.325) centre (-31.45, 58.325) ccw
  arc A84 (-32.45, -0.5741) -> (-34.4634, -2.5875) centre (-31.45, -3.5875) ccw
  line L246 (-110.1179, -34.5438) -> (-110.825, -34.5438)
  arc A85 (49.6741, 57.325) -> (55.7009, 57.325) centre (52.6875, 58.325) ccw
  arc A86 (-104.5542, -33.5438) -> (-104.5542, -35.5438) centre (-110.825, -34.5438) ccw
  arc A87 (-28.4366, 59.325) -> (-30.45, 61.3384) centre (-31.45, 58.325) ccw
  line L247 (-32.1571, 58.325) -> (-31.45, 58.325)
  line L248 (-31.45, 58.325) -> (-32.1571, 58.325)
  line L249 (-107.8116, 57.325) -> (-34.4634, 57.325)
  arc A88 (-37.7208, -4.5875) -> (-32.45, -9.8583) centre (-31.45, -3.5875) ccw
  arc A89 (55.7009, 59.325) -> (53.6875, 61.3384) centre (52.6875, 58.325) ccw
  line L250 (52.6875, 83.725) -> (52.6875, 83.0179)
  arc A90 (-34.4634, -4.5875) -> (-32.45, -6.6009) centre (-31.45, -3.5875) ccw
  line L251 (-34.4634, 28.3687) -> (-107.8116, 28.3687)
  line L252 (-109.1179, -2.5875) -> (-110.825, -2.5875)
  line L253 (53.3946, 58.325) -> (52.6875, 58.325)
  line L254 (-31.7429, -4.5875) -> (-33.1571, -4.5875)
  arc A91 (-107.8116, 28.3687) -> (-107.8116, 26.3687) centre (-110.825, 27.3687) ccw
  arc A92 (-107.8116, 28.3687) -> (-107.8116, 26.3687) centre (-110.825, 27.3687) ccw
  line L255 (-31.7429, 26.3687) -> (-33.1571, 26.3687)
  arc A93 (46.4167, 57.325) -> (58.9583, 57.325) centre (52.6875, 58.325) ccw
  arc A94 (-28.8794, 60.1885) -> (-29.5865, 60.8956) centre (-31.45, 58.325) ccw
  line L256 (135.1179, 59.325) -> (136.825, 59.325)
  arc A95 (51.6875, 61.3384) -> (50.1169, 60.1885) centre (52.6875, 58.325) ccw
  arc A96 (-29.5865, -31.9731) -> (-30.45, -31.5303) centre (-31.45, -34.5438) ccw
  arc A97 (-32.45, -62.4866) -> (-33.3135, -62.9294) centre (-31.45, -65.5) ccw
  line L257 (-29.5865, -62.9294) -> (-29.5585, -62.9014)
  line L258 (-31.8036, -34.8973) -> (-31.45, -35.2509)
  line L259 (-33.3135, -62.9294) -> (-31.45, -64.7929)
  line L260 (50.9804, 59.325) -> (52.3946, 59.325)
  arc A98 (-33.3135, 60.8956) -> (-34.4634, 59.325) centre (-31.45, 58.325) ccw
  arc A99 (-30.45, -37.5572) -> (-29.5865, -37.1144) centre (-31.45, -34.5438) ccw
  line L261 (51.6875, 60.0321) -> (51.6875, 58.6179)
  line L262 (-31.8036, -34.8973) -> (-32.1571, -34.5438)
  line L263 (-29.5865, -37.1144) -> (-29.5585, -37.1424)
  line L264 (-31.1571, 57.325) -> (-29.7429, 57.325)
  line L265 (-33.3135, -37.1144) -> (-33.3415, -37.1424)
  line L266 (-31.95, -62.8721) -> (-31.95, -37.1716)
  line L267 (-31.45, -33.8366) -> (-29.5865, -31.9731)
  line L268 (-31.45, -64.7929) -> (-28.8514, -67.3915)
  line L269 (-32.1571, -34.5438) -> (-32.45, -34.2509)
  arc A100 (51.6875, 64.5958) -> (46.4167, 59.325) centre (52.6875, 58.325) ccw
  line L270 (53.6875, 60.0321) -> (53.6875, 58.6179)
  arc A101 (-29.5865, -62.9294) -> (-30.45, -62.4866) centre (-31.45, -65.5) ccw
  line L271 (-28.4366, 59.325) -> (49.6741, 59.325)
  line L272 (53.6875, 83.725) -> (53.6875, 82.0179)
  line L273 (-107.8116, 59.325) -> (-34.4634, 59.325)
  line L274 (-28.4366, 57.325) -> (49.6741, 57.325)
  line L275 (-31.45, -35.958) -> (-30.4027, -37.0052)
  arc A102 (-31.95, -37.1716) -> (-32.4973, -37.0052) centre (-31.45, -34.5438) cw
  arc A103 (-107.8116, 59.325) -> (-107.8116, 57.325) centre (-110.825, 58.325) ccw
  line L276 (-31.1571, 59.325) -> (-29.7429, 59.325)
  line L277 (136.825, 58.325) -> (136.1179, 58.325)
  arc A104 (-107.8116, 59.325) -> (-107.8116, 57.325) centre (-110.825, 58.325) ccw
  line L278 (135.1179, 57.325) -> (136.825, 57.325)
  arc A105 (-30.95, -62.8721) -> (-30.4027, -63.0385) centre (-31.45, -65.5) cw
  line L279 (-31.45, -64.0858) -> (-32.4973, -63.0385)
  arc A106 (-34.0206, -32.6803) -> (-34.4634, -33.5438) centre (-31.45, -34.5438) ccw
  line L280 (-31.8036, -34.1902) -> (-32.1571, -34.5438)
  line L281 (-28.8514, -32.6522) -> (-31.45, -35.2509)
  arc A107 (-32.4973, -63.0385) -> (-31.95, -62.8721) centre (-31.45, -65.5) cw
  arc A108 (130.5542, 57.325) -> (130.5542, 59.325) centre (136.825, 58.325) ccw
  line L282 (-30.7429, 58.325) -> (-31.45, 58.325)
  arc A109 (-34.4634, 57.325) -> (-32.45, 55.3116) centre (-31.45, 58.325) ccw
  arc A110 (-37.7208, 57.325) -> (-32.45, 52.0542) centre (-31.45, 58.325) ccw
  arc A111 (-33.3135, -37.1144) -> (-32.45, -37.5572) centre (-31.45, -34.5438) ccw
  arc A112 (51.6875, 61.3384) -> (49.6741, 59.325) centre (52.6875, 58.325) ccw
  line L283 (-31.8036, -34.1902) -> (-31.45, -33.8366)
  line L284 (-32.1571, -34.5438) -> (-32.45, -34.8366)
  line L285 (-30.95, -37.1716) -> (-30.95, -62.8721)
  line L286 (-31.45, -64.7929) -> (-29.5865, -62.9294)
  line L287 (52.6875, 59.0321) -> (52.6875, 58.325)
  line L288 (52.6875, 58.325) -> (52.6875, 59.0321)
  arc A113 (-34.4634, -35.5438) -> (-34.0206, -36.4072) centre (-31.45, -34.5438) ccw
  line L289 (-32.4973, -37.0052) -> (-31.45, -35.958)
  line L290 (-30.4027, -63.0385) -> (-31.45, -64.0858)
  line L291 (-31.45, -35.2509) -> (-29.5865, -37.1144)
  line L292 (-31.45, -35.2509) -> (-33.3135, -37.1144)
  line L293 (-33.1571, 59.325) -> (-31.7429, 59.325)
  arc A114 (53.6875, 80.7116) -> (51.6875, 80.7116) centre (52.6875, 83.725) ccw
  arc A115 (-30.4027, -37.0052) -> (-30.95, -37.1716) centre (-31.45, -34.5438) cw
  line L294 (-33.3415, -62.9014) -> (-33.3135, -62.9294)
  arc A116 (53.6875, 77.4542) -> (51.6875, 77.4542) centre (52.6875, 83.725) ccw
  line L295 (50.9804, 57.325) -> (54.3946, 57.325)
  line L296 (-29.5865, -31.9731) -> (-29.5585, -31.9451)
  line L297 (-31.8036, -65.1464) -> (-31.45, -64.7929)
  line L298 (53.6875, 80.7116) -> (53.6875, 61.3384)
  arc A117 (-30.45, 77.4542) -> (-32.45, 77.4542) centre (-31.45, 83.725) ccw
extrude "Extrude7" add sketch "split_break_dividers" along normal blind 50.8 contours L0 A1 L11 A3 L42 L46 L69 L92 A27 L98 L113 A35 L123 L124 | A15 L54 L57 L61 L63 A20 L76 A21 L78 A24 L82 L84 L85 L88 | A23 L93 L100 L101 L102 L104 A29 A32 L111 L114 A34 L120 L121 L129 | L266 L275 A102 A105 L279 A107 L285 L289 L290 A115
equation "d2 = 10\""
equation "d55 = 2\""
equation "d85 = 2\""
named bodies: "Tray"
